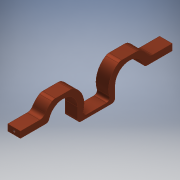
# Autodesk Inventor part: EPS_RegulatorHeatsinkBatteryAdapter
Saved by Autodesk Inventor 2018 (Build 220112000, 112)
## iProperties
Created: 2020-12-05
Part Number: EPS_RegulatorHeatsinkBatteryAdapter
Material: Copper
Document SubType Name: Modeling
Designer: Bradley
Density: 8.94 g/cm^3
Appearance: Copper - Satin
Author: Bradley
Autodesk Inventor part; units mm, degrees
ref_plane "YZ Plane" through (0, 0, 0) normal (1, 0, 0) x (0, 1, 0)
ref_plane "XZ Plane" through (0, 0, 0) normal (0, 1, 0) x (-1, 0, 0)
ref_plane "XY Plane" through (0, 0, 0) normal (0, 0, 1) x (1, 0, 0)
sketch "Sketch1" plane through (0, 0, 0) normal (1, 0, 0) x (0, 1, 0)
  line L0 (-11.75, 0.3) -> (11.75, 0.3)
  arc A0 (30.2011, 10.1) -> (11.75, 9.15) centre (21, 9.15) ccw
  arc A1 (-11.75, 9.15) -> (-30.2011, 10.1) centre (-21, 9.15) ccw
  line L1 (-30.2011, 10.1) -> (-48, 10.1)
  line L2 (-48, 10.1) -> (-48, 14.1)
  line L3 (-48, 14.1) -> (-33.2906, 14.1)
  arc A2 (-8.4379, 4.9361) -> (-33.2906, 14.1) centre (-21, 9.15) ccw
  arc A3 (33.2906, 14.1) -> (8.4379, 4.9361) centre (21, 9.15) ccw
  line L4 (30.2011, 10.1) -> (48, 10.1)
  line L5 (48, 10.1) -> (48, 14.1)
  line L6 (48, 14.1) -> (33.2906, 14.1)
  line L7 (6.5418, 2.3) -> (-6.5418, 2.3)
  line L8 (-26.9279, 21) -> (-15.0721, 21)
  line L9 (15.0721, 21) -> (26.9279, 21)
  line L10 (11.75, 9.15) -> (11.75, 0.3)
  line L11 (-11.75, 9.15) -> (-11.75, 0.3)
  arc A4 (-8.4379, 4.9361) -> (-6.5418, 2.3) centre (-6.5418, 4.3) ccw
  arc A5 (6.5418, 2.3) -> (8.4379, 4.9361) centre (6.5418, 4.3) ccw
  point P0 (0, 0)
  point P1 (0, 0.3)
  point P2 (0, 2.3)
  dimension "d1" = 9.25
  dimension "d3" = 42
  dimension "d4" = 96
  dimension "d5" = 4
  dimension "d8" = 4
  dimension "d11" = 0.3
  dimension "d13" = 10.1
  dimension "d14" = 9.15
  dimension "d15" = 21
  dimension "d26" = 2
  dimension "d30" = 2
  dimension "d31" = 13.0836
  constraints: 24 end point, 16 point on circle, 6 centre point, 6 tangent, 5 horizontal, 5 perpendicular, 3 equal length, 2 concentric, 2 equal radius, 2 midpoint, 2 point on line, 2 vertical alignment, 1 collinear, 1 horizontal alignment, 1 parallel
  measures "d1" radius of A1
  measures "d3" distance of A0.centre A1.centre
  measures "d4" distance between parallel lines of L5 L2
  measures "d5" distance of L1.end L2.end
  measures "d8" radial gap between concentric circles of A2 A1
  measures "d11" distance from line of point (0, 0) L0
  measures "d13" distance from line of point (0, 0) L1
  measures "d14" vertical distance of point (0, 0) A1.centre
  measures "d15" distance from line of point (0, 0) L8
  measures "d26" distance between parallel lines of L0 L7
  measures "d30" radius of A4
  measures "d31" distance of L7.start L7.end
extrude "Extrusion1" add sketch "Sketch1" along normal mid plane 8 contours L11 A1 L1 L2 L3 A2 L8 A4 L7 A5 A3 L9 L6 L5 L4 A0 L10 L0
sketch "Sketch2" plane through (-4, 48, 14.1) normal (0, 1, 0) x (1, 0, 0)
  line L0 (0, 0) -> (8, 0) projected
  line L1 (8, 4) -> (8, 0) projected
  line L2 (0, 4) -> (8, 4) projected
  line L3 (0, 0) -> (0, 4) projected
  line L4 (0, 4) -> (8, 4) projected
  line L5 (0, 0) -> (0, 4) projected
  point P0 (4, 14.1)
  point P1 (4, 2)
  point P2 (4, 4)
  point P3 (0, 2)
  constraints: 2 midpoint, 1 horizontal alignment, 1 vertical alignment
hole "Hole1" at (0, 48, 12.1) direction (0, -1, 0) diameter 1.567 depth 6.3 tip angle 118 thread size "M2x0.4" class "6H" standard "ANSI Metric M Profile"
mirror "Mirror1" about plane through (0, 0, 0) normal (0, 1, 0) of "Hole1"
fillet "Fillet3" radius 4 6 edges at (0, -26.9279, 21) (0, -15.0721, 21) (0, 15.0721, 21) (0, 26.9279, 21) (0, 33.2906, 14.1) (0, -33.2906, 14.1)
fillet "Fillet3" radius 2 4 edges at (0, -30.2011, 10.1) (0, 30.2011, 10.1) (0, -11.75, 0.3) (0, 11.75, 0.3)
body "Solid1"
